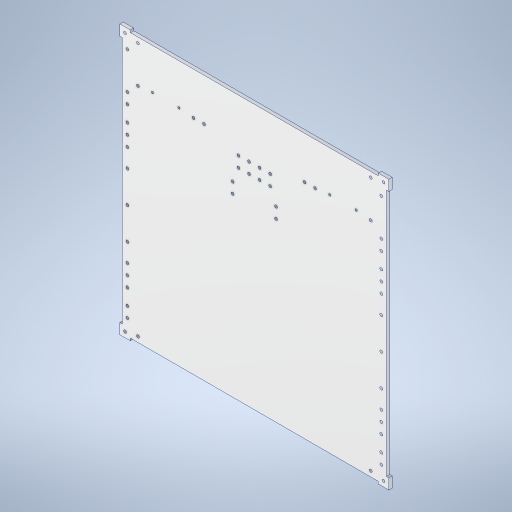
# Autodesk Inventor part: Printer Base Plate RevI
Saved by Autodesk Inventor 2024 (Build 280153000, 153)
## iProperties
Created: 2024-08-01
Part Number: Printer Base Plate RevI
Material: Aluminum 6061
Document SubType Name: Modeling
Designer: Ishaan
Density: 2.7 g/cm^3
Appearance: Aluminum - Flat
Author: Ishaan
Autodesk Inventor part; units mm, degrees
ref_plane "YZ Plane" through (0, 0, 0) normal (1, 0, 0) x (0, 1, 0)
ref_plane "XZ Plane" through (0, 0, 0) normal (0, 1, 0) x (-1, 0, 0)
ref_plane "XY Plane" through (0, 0, 0) normal (0, 0, 1) x (1, 0, 0)
sketch "Sketch1" plane through (0, 0, 0) normal (0, 0, 1) x (1, 0, 0)
  line L0 (254.35, -254.35) -> (-254.35, -254.35)
  line L1 (-254.35, -254.35) -> (-254.35, 254.35)
  line L2 (-254.35, 254.35) -> (254.35, 254.35)
  line L3 (254.35, 254.35) -> (254.35, -254.35)
  line L4 (254.35, -254.35) -> (-254.35, 254.35) construction
  line L5 (-254.35, -254.35) -> (254.35, 254.35) construction
  line L6 (-254.35, -254.35) -> (-234.35, -254.35) construction
  line L7 (-234.35, -254.35) -> (-234.35, -234.35) construction
  line L8 (-234.35, -234.35) -> (-254.35, -234.35) construction
  line L9 (-254.35, -234.35) -> (-254.35, -254.35) construction
  line L10 (-210, -250) -> (-250, -250) construction
  line L11 (-250, -250) -> (-250, -210) construction
  line L12 (-250, -210) -> (-210, -210) construction
  line L13 (-210, -210) -> (-210, -250) construction
  line L14 (-210, -250) -> (-250, -210) construction
  line L15 (-250, -250) -> (-210, -210) construction
  line L16 (-220, -240) -> (-240, -240) construction
  line L17 (-240, -240) -> (-240, -220) construction
  line L18 (-240, -220) -> (-220, -220) construction
  line L19 (-220, -220) -> (-220, -240) construction
  line L20 (-220, -240) -> (-240, -220) construction
  line L21 (-240, -240) -> (-220, -220) construction
  line L22 (254.35, -254.35) -> (234.35, -254.35) construction
  line L23 (234.35, -254.35) -> (234.35, -234.35) construction
  line L24 (234.35, -234.35) -> (254.35, -234.35) construction
  line L25 (254.35, -234.35) -> (254.35, -254.35) construction
  line L26 (210, -210) -> (250, -210) construction
  line L27 (250, -210) -> (250, -250) construction
  line L28 (250, -250) -> (210, -250) construction
  line L29 (210, -250) -> (210, -210) construction
  line L30 (210, -210) -> (250, -250) construction
  line L31 (250, -210) -> (210, -250) construction
  line L32 (240, -240) -> (220, -240) construction
  line L33 (220, -240) -> (220, -220) construction
  line L34 (220, -220) -> (240, -220) construction
  line L35 (240, -220) -> (240, -240) construction
  line L36 (240, -240) -> (220, -220) construction
  line L37 (220, -240) -> (240, -220) construction
  line L38 (-254.35, 254.35) -> (-234.35, 254.35) construction
  line L39 (-234.35, 254.35) -> (-234.35, 234.35) construction
  line L40 (-234.35, 234.35) -> (-254.35, 234.35) construction
  line L41 (-254.35, 234.35) -> (-254.35, 254.35) construction
  line L42 (254.35, 254.35) -> (234.35, 254.35) construction
  line L43 (234.35, 254.35) -> (234.35, 234.35) construction
  line L44 (234.35, 234.35) -> (254.35, 234.35) construction
  line L45 (254.35, 234.35) -> (254.35, 254.35) construction
  line L46 (210, 210) -> (250, 210) construction
  line L47 (250, 210) -> (250, 250) construction
  line L48 (250, 250) -> (210, 250) construction
  line L49 (210, 250) -> (210, 210) construction
  line L50 (210, 210) -> (250, 250) construction
  line L51 (250, 210) -> (210, 250) construction
  line L52 (240, 220) -> (220, 220) construction
  line L53 (220, 220) -> (220, 240) construction
  line L54 (220, 240) -> (240, 240) construction
  line L55 (240, 240) -> (240, 220) construction
  line L56 (240, 220) -> (220, 240) construction
  line L57 (220, 220) -> (240, 240) construction
  line L58 (-210, 210) -> (-250, 210) construction
  line L59 (-250, 210) -> (-250, 250) construction
  line L60 (-250, 250) -> (-210, 250) construction
  line L61 (-210, 250) -> (-210, 210) construction
  line L62 (-210, 210) -> (-250, 250) construction
  line L63 (-250, 210) -> (-210, 250) construction
  line L64 (-240, 220) -> (-220, 220) construction
  line L65 (-220, 220) -> (-220, 240) construction
  line L66 (-220, 240) -> (-240, 240) construction
  line L67 (-240, 240) -> (-240, 220) construction
  line L68 (-240, 220) -> (-220, 240) construction
  line L69 (-220, 220) -> (-240, 240) construction
  line L70 (250, 140) -> (210, 140) construction
  line L71 (210, 140) -> (210, 180) construction
  line L72 (210, 180) -> (250, 180) construction
  line L73 (250, 180) -> (250, 140) construction
  line L74 (250, 140) -> (210, 180) construction
  line L75 (210, 140) -> (250, 180) construction
  line L76 (240, 150) -> (220, 150) construction
  line L77 (220, 150) -> (220, 170) construction
  line L78 (220, 170) -> (240, 170) construction
  line L79 (240, 170) -> (240, 150) construction
  line L80 (240, 150) -> (220, 170) construction
  line L81 (220, 150) -> (240, 170) construction
  line L82 (-40, 161) -> (40, 161) construction
  line L83 (40, 161) -> (40, 121) construction
  line L84 (40, 121) -> (-40, 121) construction
  line L85 (-40, 121) -> (-40, 161) construction
  line L86 (-40, 161) -> (40, 121) construction
  line L87 (40, 161) -> (-40, 121) construction
  line L88 (30, 131) -> (-30, 131) construction
  line L89 (-30, 131) -> (-30, 151) construction
  line L90 (-30, 151) -> (30, 151) construction
  line L91 (30, 151) -> (30, 131) construction
  line L92 (30, 131) -> (-30, 151) construction
  line L93 (-30, 131) -> (30, 151) construction
  line L94 (10, 131) -> (-10, 131) construction
  line L95 (-10, 131) -> (-10, 151) construction
  line L96 (-10, 151) -> (10, 151) construction
  line L97 (10, 151) -> (10, 131) construction
  line L98 (10, 131) -> (-10, 151) construction
  line L99 (-10, 131) -> (10, 151) construction
  line L100 (125, 160) -> (85, 160) construction
  line L101 (85, 160) -> (85, 180) construction
  line L102 (85, 180) -> (125, 180) construction
  line L103 (125, 180) -> (125, 160) construction
  line L104 (125, 160) -> (85, 180) construction
  line L105 (85, 160) -> (125, 180) construction
  line L106 (95, 170) -> (115, 170) construction
  line L107 (-210, 140) -> (-250, 140) construction
  line L108 (-250, 140) -> (-250, 180) construction
  line L109 (-250, 180) -> (-210, 180) construction
  line L110 (-210, 180) -> (-210, 140) construction
  line L111 (-210, 140) -> (-250, 180) construction
  line L112 (-250, 140) -> (-210, 180) construction
  line L113 (-240, 150) -> (-220, 150) construction
  line L114 (-220, 150) -> (-220, 170) construction
  line L115 (-220, 170) -> (-240, 170) construction
  line L116 (-240, 170) -> (-240, 150) construction
  line L117 (-240, 150) -> (-220, 170) construction
  line L118 (-220, 150) -> (-240, 170) construction
  line L119 (-85, 160) -> (-125, 160) construction
  line L120 (-125, 160) -> (-125, 180) construction
  line L121 (-125, 180) -> (-85, 180) construction
  line L122 (-85, 180) -> (-85, 160) construction
  line L123 (-85, 160) -> (-125, 180) construction
  line L124 (-125, 160) -> (-85, 180) construction
  line L125 (-115, 170) -> (-95, 170) construction
  line L126 (-230, 50) -> (-250, 50) construction
  line L127 (-250, 50) -> (-250, 90) construction
  line L128 (-250, 90) -> (-230, 90) construction
  line L129 (-230, 90) -> (-230, 50) construction
  line L130 (-230, 50) -> (-250, 90) construction
  line L131 (-250, 50) -> (-230, 90) construction
  line L132 (-240, 60) -> (-240, 80) construction
  line L133 (250, 50) -> (230, 50) construction
  line L134 (230, 50) -> (230, 90) construction
  line L135 (230, 90) -> (250, 90) construction
  line L136 (250, 90) -> (250, 50) construction
  line L137 (250, 50) -> (230, 90) construction
  line L138 (230, 50) -> (250, 90) construction
  line L139 (240, 80) -> (240, 60) construction
  line L140 (-254.35, -234.35) -> (-234.35, -254.35) construction
  line L141 (254.35, -234.35) -> (234.35, -254.35) construction
  line L142 (234.35, 254.35) -> (254.35, 234.35) construction
  line L143 (-254.35, 234.35) -> (-234.35, 254.35) construction
  line L144 (-230, -160) -> (-250, -160) construction
  line L145 (-250, -160) -> (-250, -120) construction
  line L146 (-250, -120) -> (-230, -120) construction
  line L147 (-230, -120) -> (-230, -160) construction
  line L148 (-230, -160) -> (-250, -120) construction
  line L149 (-250, -160) -> (-230, -120) construction
  line L150 (-240, -130) -> (-240, -150) construction
  line L151 (250, -160) -> (230, -160) construction
  line L152 (230, -160) -> (230, -120) construction
  line L153 (230, -120) -> (250, -120) construction
  line L154 (250, -120) -> (250, -160) construction
  line L155 (250, -160) -> (230, -120) construction
  line L156 (230, -160) -> (250, -120) construction
  line L157 (240, -130) -> (240, -150) construction
  line L158 (-230, 50) -> (-230, -120) construction
  point P0 (0, 0)
  point P1 (-230, -230)
  point P2 (230, -230)
  point P3 (230, 230)
  point P4 (-230, 230)
  point P5 (230, 160)
  point P6 (0, 141)
  point P7 (85, 170)
  point P8 (105, 170)
  point P9 (-230, 160)
  point P10 (-105, 170)
  point P11 (-240, 70)
  point P12 (240, 70)
  point P13 (-244.35, 244.35)
  point P14 (244.35, 244.35)
  point P15 (244.35, -244.35)
  point P16 (-244.35, -244.35)
  point P17 (-240, -140)
  point P18 (240, -140)
  point P19 (-240, -120)
  point P20 (-240, 50)
  point P21 (-230, -35)
  point P22 (0, 121)
  dimension "d0" = 508.7
  dimension "d1" = 508.7
  dimension "d2" = 20
  dimension "d3" = 20
  dimension "d4" = 40
  dimension "d5" = 40
  dimension "d6" = 4.35
  dimension "d7" = 4.35
  dimension "d8" = 20
  dimension "d9" = 20
  dimension "d10" = 4.35
  dimension "d11" = 4.35
  dimension "d12" = 4.35
  dimension "d13" = 4.35
  dimension "d14" = 4.35
  dimension "d15" = 4.35
  dimension "d16" = 4.35
  dimension "d17" = 70
  dimension "d18" = 80
  dimension "d19" = 40
  dimension "d20" = 60
  dimension "d21" = 20
  dimension "d22" = 20
  dimension "d23" = 20
  dimension "d24" = 40
  dimension "d25" = 20
  dimension "d28" = 20
  dimension "d30" = 20
  dimension "d33" = 50
  dimension "d59" = 50
  dimension "d84" = 1
  dimension "d100" = 50
  dimension "d101" = 50
  dimension "d102" = 170
  dimension "d103" = 45
  dimension "d104" = 45
  dimension "d105" = 170
  dimension "d139" = 219.35
  dimension "d140" = 156
  constraints: 318 end point, 59 midpoint, 52 parallel, 40 equal length, 32 coincident, 28 horizontal, 26 perpendicular, 6 collinear, 5 vertical, 3 vertical alignment
  measures "d0" distance of L1.end L2.end
  measures "d1" distance of L0.end L1.end
  measures "d2" distance of L8.end L7.end
  measures "d3" distance of L7.end L6.end
  measures "d4" distance of L11.end L12.end
  measures "d5" distance of L10.end L11.end
  measures "d6" distance between parallel lines of L11 L1
  measures "d7" distance between parallel lines of L0 L10
  measures "d8" distance of L17.end L18.end
  measures "d9" distance of L16.end L17.end
  measures "d10" distance between parallel lines of L0 L28
  measures "d11" distance between parallel lines of L3 L27
  measures "d12" distance between parallel lines of L2 L48
  measures "d13" distance between parallel lines of L3 L47
  measures "d14" distance between parallel lines of L2 L60
  measures "d15" distance between parallel lines of L59 L1
  measures "d16" distance between parallel lines of L3 L73
  measures "d17" distance between parallel lines of L72 L48
  measures "d18" distance of L83.end L84.end
  measures "d19" distance of L82.end L83.end
  measures "d20" distance of L89.end L90.end
  measures "d21" distance of L88.end L89.end
  measures "d22" distance of L95.end L96.end
  measures "d23" distance of L94.end L95.end
  measures "d24" distance of L101.end L102.end
  measures "d25" distance of L100.end L101.end
  measures "d28" distance of L106.start L106.end
  measures "d30" distance of L125.start L125.end
  measures "d33" distance between parallel lines of L70 L135
  measures "d59" distance between parallel lines of L128 L107
  measures "d84" distance between parallel lines of L82 L119
  measures "d100" distance between parallel lines of L12 L144
  measures "d101" distance between parallel lines of L151 L26
  measures "d102" distance of point (-240, -120) point (-240, 50)
  measures "d103" distance between parallel lines of L85 L122
  measures "d104" distance between parallel lines of L101 L83
  measures "d105" distance from line of L101.end L122
  measures "d139" distance from line of L0 point (-230, -35)
  measures "d140" vertical distance of point (0, 121) point (-230, -35)
extrude "Extrusion1" add sketch "Sketch1" along normal blind 6.35
hole "Hole1" at (-240, -220, 0) at (-220, -240, 0) at (220, -240, 0) at (240, -220, 0) at (220, 240, 0) at (240, 220, 0) at (-240, 220, 0) at (-220, 240, 0) at (220, 170, 0) at (240, 150, 0) at (-30, 151, 0) at (-30, 131, 0) at (-10, 151, 0) at (-10, 131, 0) at (10, 151, 0) at (10, 131, 0) at (30, 151, 0) at (30, 131, 0) at (95, 170, 0) at (115, 170, 0) at (-220, 170, 0) at (-240, 150, 0) at (-115, 170, 0) at (-95, 170, 0) at (-240, 80, 0) at (-240, 60, 0) at (240, 80, 0) at (240, 60, 0) at (-244.35, 244.35, 0) at (244.35, 244.35, 0) at (244.35, -244.35, 0) at (-244.35, -244.35, 0) at (-240, -130, 0) at (-240, -150, 0) at (240, -130, 0) at (240, -150, 0) direction (0, 0, 1) diameter 5.3 end through all
sketch "Sketch3" plane through (0, 0, 0) normal (0, 0, -1) x (-1, 0, 0)
  line L0 (41, 83) -> (-41, 83) construction
  line L1 (-41, 83) -> (-41, 103) construction
  line L2 (-41, 103) -> (41, 103) construction
  line L3 (41, 103) -> (41, 83) construction
  line L4 (41, 83) -> (-41, 103) construction
  line L5 (-41, 83) -> (41, 103) construction
  line L6 (27, 66) -> (-27, 66) construction
  line L7 (-27, 66) -> (-27, 120) construction
  line L8 (-27, 120) -> (27, 120) construction
  line L9 (27, 120) -> (27, 66) construction
  line L10 (27, 66) -> (-27, 120) construction
  line L11 (-27, 66) -> (27, 120) construction
  line L12 (-40, 121) -> (40, 121) construction
  point P0 (0, 0)
  point P1 (0, 93)
  point P2 (0, 121)
  dimension "d43" = 82
  dimension "d44" = 20
  dimension "d45" = 54
  dimension "d46" = 54
  dimension "d47" = 1
  dimension "d48" = 28
  constraints: 24 end point, 5 midpoint, 4 coincident, 4 parallel, 2 horizontal, 2 perpendicular, 1 vertical alignment
  measures "d43" distance of L1.end L2.end
  measures "d44" distance of L0.end L1.end
  measures "d45" distance of L7.end L8.end
  measures "d46" distance of L6.end L7.end
  measures "d47" distance between parallel lines of L8 L12
  measures "d48" distance from line of point (0, 93) L12
hole "Hole2" at (41, 103, 0) at (41, 83, 0) at (-41, 103, 0) at (-41, 83, 0) direction (0, 0, 1) diameter 5.3 end through all
sketch "Sketch4" plane through (0, 0, 6.35) normal (0, 0, 1) x (1, 0, 0)
  line L0 (235, -224.35) -> (-235, -224.35) construction
  line L1 (-235, -224.35) -> (-235, 10.65) construction
  line L2 (-235, 10.65) -> (235, 10.65) construction
  line L3 (235, 10.65) -> (235, -224.35) construction
  line L4 (235, -224.35) -> (-235, 10.65) construction
  line L5 (-235, -224.35) -> (235, 10.65) construction
  circle A0 centre (-41, 83) radius 2.65 construction
  circle A1 centre (-41, 103) radius 2.65 construction
  circle A2 centre (41, 83) radius 2.65 construction
  circle A3 centre (41, 103) radius 2.65 construction
  circle A4 centre (-244.35, -244.35) radius 2.65 construction
  circle A5 centre (244.35, -244.35) radius 2.65 construction
  circle A6 centre (244.35, 244.35) radius 2.65 construction
  circle A7 centre (-244.35, 244.35) radius 2.65 construction
  circle A8 centre (240, 60) radius 2.65 construction
  circle A9 centre (240, 80) radius 2.65 construction
  circle A10 centre (-240, 60) radius 2.65 construction
  circle A11 centre (-240, 80) radius 2.65 construction
  circle A12 centre (-95, 170) radius 2.65 construction
  circle A13 centre (-115, 170) radius 2.65 construction
  circle A14 centre (-240, 150) radius 2.65 construction
  circle A15 centre (-220, 170) radius 2.65 construction
  circle A16 centre (115, 170) radius 2.65 construction
  circle A17 centre (95, 170) radius 2.65 construction
  circle A18 centre (30, 131) radius 2.65 construction
  circle A19 centre (30, 151) radius 2.65 construction
  circle A20 centre (10, 131) radius 2.65 construction
  circle A21 centre (10, 151) radius 2.65 construction
  circle A22 centre (-10, 131) radius 2.65 construction
  circle A23 centre (-10, 151) radius 2.65 construction
  circle A24 centre (-30, 131) radius 2.65 construction
  circle A25 centre (-30, 151) radius 2.65 construction
  circle A26 centre (240, 150) radius 2.65 construction
  circle A27 centre (220, 170) radius 2.65 construction
  circle A28 centre (-220, 240) radius 2.65 construction
  circle A29 centre (-240, 220) radius 2.65 construction
  circle A30 centre (240, 220) radius 2.65 construction
  circle A31 centre (220, 240) radius 2.65 construction
  circle A32 centre (240, -220) radius 2.65 construction
  circle A33 centre (220, -240) radius 2.65 construction
  circle A34 centre (-220, -240) radius 2.65 construction
  circle A35 centre (-240, -220) radius 2.65 construction
  line L6 (254.35, 254.35) -> (-254.35, 254.35) construction
  line L7 (-254.35, 254.35) -> (-254.35, -254.35) construction
  line L8 (-254.35, -254.35) -> (254.35, -254.35) construction
  line L9 (254.35, -254.35) -> (254.35, 254.35) construction
  circle A36 centre (-117.5, -106.85) radius 117.5 construction
  circle A37 centre (117.5, -106.85) radius 117.5 construction
  circle A38 centre (-117.5, -106.85) radius 21.75 construction
  circle A39 centre (117.5, -106.85) radius 21.75 construction
  line L10 (-117.5, -85.1) -> (-98.6639, -95.975) construction
  line L11 (-98.6639, -95.975) -> (-98.6639, -117.725) construction
  line L12 (-98.6639, -117.725) -> (-117.5, -128.6) construction
  line L13 (-117.5, -128.6) -> (-136.3361, -117.725) construction
  line L14 (-136.3361, -117.725) -> (-136.3361, -95.975) construction
  line L15 (-136.3361, -95.975) -> (-117.5, -85.1) construction
  line L16 (117.5, -85.1) -> (136.3361, -95.975) construction
  line L17 (136.3361, -95.975) -> (136.3361, -117.725) construction
  line L18 (136.3361, -117.725) -> (117.5, -128.6) construction
  line L19 (117.5, -128.6) -> (98.6639, -117.725) construction
  line L20 (98.6639, -117.725) -> (98.6639, -95.975) construction
  line L21 (98.6639, -95.975) -> (117.5, -85.1) construction
  point P0 (0, 0)
  point P1 (0, -106.85)
  point P2 (0, 10.65)
  dimension "d66" = 43.5
  dimension "d67" = 43.5
  dimension "d60" = 30
  dimension "d63" = 235
  dimension "d65" = 470
  constraints: 36 end point, 16 coincident, 3 midpoint, 3 tangent, 3 vertical alignment, 2 centre point, 2 horizontal alignment, 2 parallel, 2 vertical, 1 equal radius, 1 horizontal, 1 perpendicular, 30 other
  measures "d60" distance between parallel lines of L0 L8
  measures "d63" distance of L0.end L1.end
  measures "d65" distance of L1.end L2.end
hole "Hole3" [suppressed]
sketch "Sketch5" plane through (0, 0, 6.35) normal (0, 0, 1) x (1, 0, 0)
  circle A0 centre (-41, 83) radius 2.65 projected
  circle A1 centre (-41, 103) radius 2.65 projected
  circle A2 centre (41, 83) radius 2.65 projected
  circle A3 centre (41, 103) radius 2.65 projected
  circle A4 centre (-244.35, -244.35) radius 2.65 projected
  circle A5 centre (244.35, -244.35) radius 2.65 projected
  circle A6 centre (244.35, 244.35) radius 2.65 projected
  circle A7 centre (-244.35, 244.35) radius 2.65 projected
  circle A8 centre (240, 60) radius 2.65 projected
  circle A9 centre (240, 80) radius 2.65 projected
  circle A10 centre (-240, 60) radius 2.65 projected
  circle A11 centre (-240, 80) radius 2.65 projected
  circle A12 centre (-95, 170) radius 2.65 projected
  circle A13 centre (-115, 170) radius 2.65 projected
  circle A14 centre (-240, 150) radius 2.65 projected
  circle A15 centre (-220, 170) radius 2.65 projected
  circle A16 centre (115, 170) radius 2.65 projected
  circle A17 centre (95, 170) radius 2.65 projected
  circle A18 centre (30, 131) radius 2.65 projected
  circle A19 centre (30, 151) radius 2.65 projected
  circle A20 centre (10, 131) radius 2.65 projected
  circle A21 centre (10, 151) radius 2.65 projected
  circle A22 centre (-10, 131) radius 2.65 projected
  circle A23 centre (-10, 151) radius 2.65 projected
  circle A24 centre (-30, 131) radius 2.65 projected
  circle A25 centre (-30, 151) radius 2.65 projected
  circle A26 centre (240, 150) radius 2.65 projected
  circle A27 centre (220, 170) radius 2.65 projected
  circle A28 centre (-220, 240) radius 2.65 projected
  circle A29 centre (-240, 220) radius 2.65 projected
  circle A30 centre (240, 220) radius 2.65 projected
  circle A31 centre (220, 240) radius 2.65 projected
  circle A32 centre (240, -220) radius 2.65 projected
  circle A33 centre (220, -240) radius 2.65 projected
  circle A34 centre (-220, -240) radius 2.65 projected
  circle A35 centre (-240, -220) radius 2.65 projected
  line L0 (254.35, 254.35) -> (-254.35, 254.35) projected
  line L1 (-254.35, 254.35) -> (-254.35, -254.35) projected
  line L2 (-254.35, -254.35) -> (254.35, -254.35) projected
  line L3 (254.35, -254.35) -> (254.35, 254.35) projected
  line L4 (-220, 170) -> (-115, 170) construction
  line L5 (115, 170) -> (220, 170) construction
  line L6 (142.5, 173) -> (192.5, 173) construction
  line L7 (-192.5, 173) -> (-142.5, 173) construction
  point P0 (0, 0)
  point P1 (167.5, 173)
  point P2 (167.5, 170)
  point P3 (-167.5, 173)
  point P4 (-167.5, 170)
  dimension "d75" = 50
  dimension "d76" = 3
  constraints: 8 end point, 4 coincident, 4 horizontal, 4 midpoint, 2 collinear, 2 vertical alignment
  measures "d75" distance of L6.start L6.end
  measures "d76" distance between parallel lines of L5 L6
hole "Hole4" at (142.5, 173, 6.35) at (192.5, 173, 6.35) at (-192.5, 173, 6.35) at (-142.5, 173, 6.35) direction (0, 0, -1) diameter 4.134 end through all thread size "M5x0.8" class "6H" standard "ANSI Metric M Profile"
sketch "Sketch6" plane through (0, 0, 6.35) normal (0, 0, 1) x (1, 0, 0)
  line L0 (-219.5, -171.85) -> (-231.5, -171.85) construction
  line L1 (-231.5, -171.85) -> (-231.5, -41.85) construction
  line L2 (-231.5, -41.85) -> (-219.5, -41.85) construction
  line L3 (-219.5, -41.85) -> (-219.5, -171.85) construction
  line L4 (-219.5, -171.85) -> (-231.5, -41.85) construction
  line L5 (-231.5, -171.85) -> (-219.5, -41.85) construction
  circle A0 centre (-117.5, -106.85) radius 116 construction
  point P0 (0, 0)
  point P1 (-225.5, -106.85)
  point P2 (-219.5, -106.85)
  point P3 (-97.5, -221.1129)
  dimension "d88" = 232
  dimension "d85" = 12
  dimension "d86" = 130
  dimension "d87" = 102
  dimension "d89" = 20
  constraints: 12 end point, 3 coincident, 3 midpoint, 2 parallel, 1 horizontal, 1 horizontal alignment, 1 perpendicular, 3 other
  measures "d85" distance between parallel lines of L3 L1
  measures "d86" distance of L0.end L1.end
  measures "d87" distance from line of point (-117.5, -106.85) L3
  measures "d89" horizontal distance of point (-117.5, -106.85) point (-97.5, -221.113)
hole "Hole5" [suppressed]
mirror "Mirror1" [suppressed]
sketch "Sketch7" plane through (0, 0, 6.35) normal (0, 0, 1) x (1, 0, 0)
  circle A0 centre (-142.5, 173) radius 2.067 projected
  circle A1 centre (-192.5, 173) radius 2.067 projected
  circle A2 centre (192.5, 173) radius 2.067 projected
  circle A3 centre (142.5, 173) radius 2.067 projected
  circle A4 centre (-41, 83) radius 2.65 projected
  circle A5 centre (-41, 103) radius 2.65 projected
  circle A6 centre (41, 83) radius 2.65 projected
  circle A7 centre (41, 103) radius 2.65 projected
  circle A8 centre (240, -150) radius 2.65 projected
  circle A9 centre (240, -130) radius 2.65 projected
  circle A10 centre (-240, -150) radius 2.65 projected
  circle A11 centre (-240, -130) radius 2.65 projected
  circle A12 centre (-244.35, -244.35) radius 2.65 projected
  circle A13 centre (244.35, -244.35) radius 2.65 projected
  circle A14 centre (244.35, 244.35) radius 2.65 projected
  circle A15 centre (-244.35, 244.35) radius 2.65 projected
  circle A16 centre (240, 60) radius 2.65 projected
  circle A17 centre (240, 80) radius 2.65 projected
  circle A18 centre (-240, 60) radius 2.65 projected
  circle A19 centre (-240, 80) radius 2.65 projected
  circle A20 centre (-95, 170) radius 2.65 projected
  circle A21 centre (-115, 170) radius 2.65 projected
  circle A22 centre (-240, 150) radius 2.65 projected
  circle A23 centre (-220, 170) radius 2.65 projected
  circle A24 centre (115, 170) radius 2.65 projected
  circle A25 centre (95, 170) radius 2.65 projected
  circle A26 centre (30, 131) radius 2.65 projected
  circle A27 centre (30, 151) radius 2.65 projected
  circle A28 centre (10, 131) radius 2.65 projected
  circle A29 centre (10, 151) radius 2.65 projected
  circle A30 centre (-10, 131) radius 2.65 projected
  circle A31 centre (-10, 151) radius 2.65 projected
  circle A32 centre (-30, 131) radius 2.65 projected
  circle A33 centre (-30, 151) radius 2.65 projected
  circle A34 centre (240, 150) radius 2.65 projected
  circle A35 centre (220, 170) radius 2.65 projected
  circle A36 centre (-220, 240) radius 2.65 projected
  circle A37 centre (-240, 220) radius 2.65 projected
  circle A38 centre (240, 220) radius 2.65 projected
  circle A39 centre (220, 240) radius 2.65 projected
  circle A40 centre (240, -220) radius 2.65 projected
  circle A41 centre (220, -240) radius 2.65 projected
  circle A42 centre (-220, -240) radius 2.65 projected
  circle A43 centre (-240, -220) radius 2.65 projected
  line L0 (254.35, 254.35) -> (-254.35, 254.35) projected
  line L1 (-254.35, 254.35) -> (-254.35, -254.35) projected
  line L2 (-254.35, -254.35) -> (254.35, -254.35) projected
  line L3 (254.35, -254.35) -> (254.35, 254.35) projected
  line L4 (-240, 150) -> (-240, 80) construction
  line L5 (-240, 130) -> (-240, 100) construction
  line L6 (-240, -150) -> (-240, -220) construction
  line L7 (-240, -170) -> (-240, -200) construction
  line L8 (240, -150) -> (240, -220) construction
  line L9 (240, -170) -> (240, -200) construction
  line L10 (240, 150) -> (240, 80) construction
  line L11 (240, 130) -> (240, 100) construction
  point P0 (0, 0)
  point P1 (-240, 115)
  point P2 (-240, -185)
  point P3 (240, -185)
  point P4 (240, 115)
  dimension "d106" = 30
  dimension "d107" = 30
  dimension "d108" = 30
  dimension "d109" = 30
  constraints: 16 end point, 8 coincident, 8 midpoint, 7 vertical, 1 parallel
  measures "d106" distance of L5.start L5.end
  measures "d107" distance of L7.start L7.end
  measures "d108" distance of L9.start L9.end
  measures "d109" distance of L11.start L11.end
hole "Hole6" at (-240, 130, 6.35) at (-240, 100, 6.35) at (-240, -170, 6.35) at (-240, -200, 6.35) at (240, -170, 6.35) at (240, -200, 6.35) at (240, 130, 6.35) at (240, 100, 6.35) direction (0, 0, -1) diameter 5.4 end through all
sketch "Sketch8" plane through (0, 0, 6.35) normal (0, 0, 1) x (1, 0, 0)
  circle A0 centre (240, 100) radius 2.7 projected
  circle A1 centre (240, 130) radius 2.7 projected
  circle A2 centre (240, -200) radius 2.7 projected
  circle A3 centre (240, -170) radius 2.7 projected
  circle A4 centre (-240, -200) radius 2.7 projected
  circle A5 centre (-240, -170) radius 2.7 projected
  circle A6 centre (-240, 100) radius 2.7 projected
  circle A7 centre (-240, 130) radius 2.7 projected
  circle A8 centre (-142.5, 173) radius 2.067 projected
  circle A9 centre (-192.5, 173) radius 2.067 projected
  circle A10 centre (192.5, 173) radius 2.067 projected
  circle A11 centre (142.5, 173) radius 2.067 projected
  circle A12 centre (-41, 83) radius 2.65 projected
  circle A13 centre (-41, 103) radius 2.65 projected
  circle A14 centre (41, 83) radius 2.65 projected
  circle A15 centre (41, 103) radius 2.65 projected
  circle A16 centre (240, -150) radius 2.65 projected
  circle A17 centre (240, -130) radius 2.65 projected
  circle A18 centre (-240, -150) radius 2.65 projected
  circle A19 centre (-240, -130) radius 2.65 projected
  circle A20 centre (-244.35, -244.35) radius 2.65 projected
  circle A21 centre (244.35, -244.35) radius 2.65 projected
  circle A22 centre (244.35, 244.35) radius 2.65 projected
  circle A23 centre (-244.35, 244.35) radius 2.65 projected
  circle A24 centre (240, 60) radius 2.65 projected
  circle A25 centre (240, 80) radius 2.65 projected
  circle A26 centre (-240, 60) radius 2.65 projected
  circle A27 centre (-240, 80) radius 2.65 projected
  circle A28 centre (-95, 170) radius 2.65 projected
  circle A29 centre (-115, 170) radius 2.65 projected
  circle A30 centre (-240, 150) radius 2.65 projected
  circle A31 centre (-220, 170) radius 2.65 projected
  circle A32 centre (115, 170) radius 2.65 projected
  circle A33 centre (95, 170) radius 2.65 projected
  circle A34 centre (30, 131) radius 2.65 projected
  circle A35 centre (30, 151) radius 2.65 projected
  circle A36 centre (10, 131) radius 2.65 projected
  circle A37 centre (10, 151) radius 2.65 projected
  circle A38 centre (-10, 131) radius 2.65 projected
  circle A39 centre (-10, 151) radius 2.65 projected
  circle A40 centre (-30, 131) radius 2.65 projected
  circle A41 centre (-30, 151) radius 2.65 projected
  circle A42 centre (240, 150) radius 2.65 projected
  circle A43 centre (220, 170) radius 2.65 projected
  circle A44 centre (-220, 240) radius 2.65 projected
  circle A45 centre (-240, 220) radius 2.65 projected
  circle A46 centre (240, 220) radius 2.65 projected
  circle A47 centre (220, 240) radius 2.65 projected
  circle A48 centre (240, -220) radius 2.65 projected
  circle A49 centre (220, -240) radius 2.65 projected
  circle A50 centre (-220, -240) radius 2.65 projected
  circle A51 centre (-240, -220) radius 2.65 projected
  line L0 (254.35, 254.35) -> (-254.35, 254.35) projected
  line L1 (-254.35, 254.35) -> (-254.35, -254.35) projected
  line L2 (-254.35, -254.35) -> (254.35, -254.35) projected
  line L3 (254.35, -254.35) -> (254.35, 254.35) projected
  line L4 (-240, -130) -> (-240, 60) construction
  line L5 (240, -130) -> (240, 60) construction
  line L6 (-240, 25) -> (-240, -95) construction
  line L7 (240, 25) -> (240, -95) construction
  point P0 (0, 0)
  point P1 (240, -35)
  point P2 (-240, -35)
  dimension "d117" = 120
  dimension "d118" = 120
  constraints: 8 end point, 4 coincident, 4 midpoint, 3 vertical, 1 parallel
  measures "d117" distance of L6.start L6.end
  measures "d118" distance of L7.start L7.end
hole "Hole7" at (240, 25, 6.35) at (240, -95, 6.35) at (-240, -95, 6.35) at (-240, 25, 6.35) at (240, -35, 6.35) at (-240, -35, 6.35) direction (0, 0, -1) diameter 5.4 end through all
sketch "Sketch9" plane through (0, 0, 6.35) normal (0, 0, 1) x (1, 0, 0)
  circle A0 centre (-240, -35) radius 2.7 projected
  circle A1 centre (240, -35) radius 2.7 projected
  circle A2 centre (-240, 25) radius 2.7 projected
  circle A3 centre (-240, -95) radius 2.7 projected
  circle A4 centre (240, -95) radius 2.7 projected
  circle A5 centre (240, 25) radius 2.7 projected
  circle A6 centre (240, 100) radius 2.7 projected
  circle A7 centre (240, 130) radius 2.7 projected
  circle A8 centre (240, -200) radius 2.7 projected
  circle A9 centre (240, -170) radius 2.7 projected
  circle A10 centre (-240, -200) radius 2.7 projected
  circle A11 centre (-240, -170) radius 2.7 projected
  circle A12 centre (-240, 100) radius 2.7 projected
  circle A13 centre (-240, 130) radius 2.7 projected
  circle A14 centre (-142.5, 173) radius 2.067 projected
  circle A15 centre (-192.5, 173) radius 2.067 projected
  circle A16 centre (192.5, 173) radius 2.067 projected
  circle A17 centre (142.5, 173) radius 2.067 projected
  circle A18 centre (-41, 83) radius 2.65 projected
  circle A19 centre (-41, 103) radius 2.65 projected
  circle A20 centre (41, 83) radius 2.65 projected
  circle A21 centre (41, 103) radius 2.65 projected
  circle A22 centre (240, -150) radius 2.65 projected
  circle A23 centre (240, -130) radius 2.65 projected
  circle A24 centre (-240, -150) radius 2.65 projected
  circle A25 centre (-240, -130) radius 2.65 projected
  circle A26 centre (-244.35, -244.35) radius 2.65 projected
  circle A27 centre (244.35, -244.35) radius 2.65 projected
  circle A28 centre (244.35, 244.35) radius 2.65 projected
  circle A29 centre (-244.35, 244.35) radius 2.65 projected
  circle A30 centre (240, 60) radius 2.65 projected
  circle A31 centre (240, 80) radius 2.65 projected
  circle A32 centre (-240, 60) radius 2.65 projected
  circle A33 centre (-240, 80) radius 2.65 projected
  circle A34 centre (-95, 170) radius 2.65 projected
  circle A35 centre (-115, 170) radius 2.65 projected
  circle A36 centre (-240, 150) radius 2.65 projected
  circle A37 centre (-220, 170) radius 2.65 projected
  circle A38 centre (115, 170) radius 2.65 projected
  circle A39 centre (95, 170) radius 2.65 projected
  circle A40 centre (30, 131) radius 2.65 projected
  circle A41 centre (30, 151) radius 2.65 projected
  circle A42 centre (10, 131) radius 2.65 projected
  circle A43 centre (10, 151) radius 2.65 projected
  circle A44 centre (-10, 131) radius 2.65 projected
  circle A45 centre (-10, 151) radius 2.65 projected
  circle A46 centre (-30, 131) radius 2.65 projected
  circle A47 centre (-30, 151) radius 2.65 projected
  circle A48 centre (240, 150) radius 2.65 projected
  circle A49 centre (220, 170) radius 2.65 projected
  circle A50 centre (-220, 240) radius 2.65 projected
  circle A51 centre (-240, 220) radius 2.65 projected
  circle A52 centre (240, 220) radius 2.65 projected
  circle A53 centre (220, 240) radius 2.65 projected
  circle A54 centre (240, -220) radius 2.65 projected
  circle A55 centre (220, -240) radius 2.65 projected
  circle A56 centre (-220, -240) radius 2.65 projected
  circle A57 centre (-240, -220) radius 2.65 projected
  line L0 (254.35, 254.35) -> (-254.35, 254.35) projected
  line L1 (-254.35, 254.35) -> (-254.35, -254.35) projected
  line L2 (-254.35, -254.35) -> (254.35, -254.35) projected
  line L3 (254.35, -254.35) -> (254.35, 254.35) projected
  line L4 (-254.35, 254.35) -> (-234.35, 254.35)
  line L5 (-234.35, 254.35) -> (-234.35, 234.35)
  line L6 (-234.35, 234.35) -> (-254.35, 234.35)
  line L7 (-254.35, 234.35) -> (-254.35, 254.35)
  line L8 (254.35, 254.35) -> (234.35, 254.35)
  line L9 (234.35, 254.35) -> (234.35, 234.35)
  line L10 (234.35, 234.35) -> (254.35, 234.35)
  line L11 (254.35, 234.35) -> (254.35, 254.35)
  line L12 (254.35, -254.35) -> (234.35, -254.35)
  line L13 (234.35, -254.35) -> (234.35, -234.35)
  line L14 (234.35, -234.35) -> (254.35, -234.35)
  line L15 (254.35, -234.35) -> (254.35, -254.35)
  line L16 (-254.35, -254.35) -> (-234.35, -254.35)
  line L17 (-234.35, -254.35) -> (-234.35, -234.35)
  line L18 (-234.35, -234.35) -> (-254.35, -234.35)
  line L19 (-254.35, -234.35) -> (-254.35, -254.35)
  line L20 (250, -250) -> (-250, -250)
  line L21 (-250, -250) -> (-250, 250)
  line L22 (-250, 250) -> (250, 250)
  line L23 (250, 250) -> (250, -250)
  line L24 (250, -250) -> (-250, 250) construction
  line L25 (-250, -250) -> (250, 250) construction
  point P0 (0, 0)
  point P1 (-250, -234.35)
  point P2 (-250, 234.35)
  point P3 (234.35, -250)
  point P4 (-234.35, -250)
  point P5 (250, 234.35)
  point P6 (250, -234.35)
  point P7 (-234.35, 250)
  point P8 (234.35, 250)
  dimension "d132" = 20
  dimension "d135" = 10
  dimension "d136" = 10
  constraints: 44 end point, 10 parallel, 7 equal length, 5 horizontal, 5 perpendicular, 2 midpoint
  measures "d132" distance of L18.end L17.end
  measures "d135" distance from line of L22 A50.centre
  measures "d136" distance from line of A51.centre L21
extrude "Extrusion2" cut sketch "Sketch9" against normal through all contours L9 L22 L5 L0 | L3 L14 L23 L10 | L6 L21 L18 L1 | L2 L17 L20 L13
equation "\"d10\" = d7"
equation "\"d11\" = d6"
equation "\"d12\" = d10"
equation "\"d13\" = d11"
equation "\"d14\" = d12"
equation "\"d15\" = d13"
equation "\"d16\" = d13"
equation "\"d33\" = d59"
equation "\"d100\" = d59"
equation "\"d67\" = d66"
equation "\"d63\" = 0.5 * d65"
body "Solid1"
